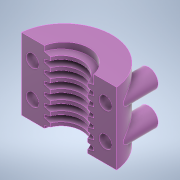
# Autodesk Inventor part: SpindleAdaptor_B_V2
Saved by Autodesk Inventor 2022.2 (Build 262287000, 287)
## iProperties
Created: 2022-11-20
Part Number: SpindleAdaptor_B_V2
Material: ABS Plastic
Document SubType Name: Modeling
Designer: jaege
Density: 1.06 g/cm^3
Appearance: Smooth - Purple
Mass: 4.16051 g
Surface Area: 27.1261 cm^2
Volume: 4.16051 cm^3
Author: jaege
Autodesk Inventor part; units mm, degrees
ref_plane "YZ Plane" through (0, 0, 0) normal (1, 0, 0) x (0, 1, 0)
ref_plane "XZ Plane" through (0, 0, 0) normal (0, 1, 0) x (-1, 0, 0)
ref_plane "XY Plane" through (0, 0, 0) normal (0, 0, 1) x (1, 0, 0)
sketch "Sketch1" plane through (0, 0, 0) normal (0, 1, 0) x (-1, 0, 0)
  circle A0 centre (0, 0) radius 10
  dimension "d0" = 20
  constraints: 1 centre point, 1 coincident
  measures "d0" diameter of A0
extrude "Extrusion1" add sketch "Sketch1" along normal blind 30
sketch "Sketch2" plane through (0, 30, 0) normal (0, 1, 0) x (1, 0, 0)
  circle A0 centre (0, 0) radius 5.25
  dimension "d3" = 10.5
  constraints: 1 centre point, 1 coincident
  measures "d3" diameter of A0
extrude "Extrusion2" cut sketch "Sketch2" against normal blind 15
sketch "Sketch3" plane through (0, 0, 0) normal (0, 0, 1) x (1, 0, 0)
  line L0 (10, 30) -> (-10, 30) projected
  line L1 (10, 0) -> (-10, 0) projected
  line L2 (-5.25, 15) -> (5.25, 15) projected
  line L3 (-5.25, 30) -> (5.25, 30) projected
  line L4 (-5.25, 30) -> (-5.25, 15) projected
  line L5 (5.25, 30) -> (5.25, 15) construction
  line L6 (-5.25, 15) -> (5.25, 15) projected
  line L7 (-4, 15) -> (4, 15) construction
  line L8 (4, 15) -> (4, 30) construction
  line L9 (4, 30) -> (-4, 30) construction
  line L10 (-4, 30) -> (-4, 15) construction
  line L11 (5.25, 30) -> (4, 29.6651)
  line L12 (2.634, 29.299) -> (4, 28.933) construction
  line L13 (4, 29.6651) -> (4, 28.933)
  line L14 (5.25, 28.5981) -> (5.25, 28)
  line L15 (5.25, 28) -> (4, 27.6651)
  line L16 (2.634, 27.299) -> (4, 26.933) construction
  line L17 (4, 29.6651) -> (2.634, 29.299) construction
  line L18 (4, 27.6651) -> (2.634, 27.299) construction
  line L19 (4, 28.933) -> (5.25, 28.5981)
  line L20 (4, 26.933) -> (5.25, 26.5981)
  line L21 (4, 27.6651) -> (4, 26.933)
  line L22 (5.25, 30) -> (5.25, 28.5981)
  line L23 (0, 30) -> (0, 15)
  point P0 (0, 0)
  point P1 (4, 29.299)
  dimension "d6" = 8
  dimension "d7" = 30
  dimension "d8" = 30
  dimension "d9" = 1.25
  dimension "d10" = 105
  dimension "d11" = 105
  dimension "d12" = 0.732
  dimension "d13" = 0.5981
  constraints: 34 end point, 9 point on line, 6 collinear, 3 midpoint, 2 parallel, 2 vertical, 1 horizontal, 1 perpendicular, 1 vertical alignment
  measures "d6" distance between parallel lines of L8 L10
  measures "d7" angle of L12 L11
  measures "d8" angle of L16 L15
  measures "d9" distance between parallel lines of L5 L13
  measures "d10" angle of L5 L11
  measures "d11" angle of L14 L15
  measures "d12" distance of L13.start L12.end
  measures "d13" distance of L14.start L14.end
coil "Coil1" sketch "Sketch3" operation add axis through (0, 30, 0) along (0, -1, 0) pitch 2 turns 7 hand right contours L22 L19 L13 L11
sketch "Sketch4" plane through (0, 0, 0) normal (0, -1, 0) x (1, 0, 0)
  circle A0 centre (0, 0) radius 2
  line L0 (-2, -2) -> (2, -2)
  line L1 (2, -2) -> (2, 1.5)
  line L2 (2, 1.5) -> (-2, 1.5)
  line L3 (-2, 1.5) -> (-2, -2)
  point P0 (1.3229, 1.5)
  point P1 (-1.3229, 1.5)
  dimension "d22" = 4
  dimension "d23" = 3.5
  constraints: 8 end point, 3 tangent, 2 parallel, 1 centre point, 1 coincident, 1 horizontal, 1 perpendicular
  measures "d22" diameter of A0
  measures "d23" distance of L0.end L1.end
extrude "Extrusion3" cut sketch "Sketch4" against normal blind 10 contours A0 L2 picked at (0.2249, -0.4939)
sketch "Sketch5" plane through (0, 0, 0) normal (0, 0, 1) x (1, 0, 0)
  line L0 (10, 30) -> (-10, 30) projected
  line L1 (-5.25, 15) -> (5.25, 15) projected
  line L2 (0, -6) -> (0, 36) projected
  line L3 (-7.625, 26) -> (-10, 26) construction
  line L4 (-7.625, 26) -> (-5.25, 26) construction
  line L5 (-5.25, 30) -> (-5.25, 15) projected
  line L6 (-10, 0) -> (-10, 30) projected
  circle A0 centre (-7.625, 19) radius 1.3375
  circle A1 centre (-7.625, 26) radius 1.3375
  circle A2 centre (7.625, 26) radius 1.3375
  circle A3 centre (7.625, 19) radius 1.3375
  point P0 (0, 0)
  point P1 (1.5921, 15)
  dimension "d26" = 4
  dimension "d27" = 4
  dimension "d28" = 2.675
  constraints: 4 centre point, 4 coincident, 4 end point, 4 vertical alignment, 3 equal radius, 2 horizontal, 2 horizontal alignment, 1 collinear, 1 symmetric about line
  measures "d26" distance from line of L0 L3.start
  measures "d27" distance from line of L1 point (-7.625, 19)
  measures "d28" diameter of A0
extrude "Extrusion4" cut sketch "Sketch5" along normal through all both and the other way through all contours A0 | A1 | A2 | A3
ref_plane "Work Plane1" through (0, 0, -10) normal (0, 0, -1) x (-1, 0, 0)
sketch "Sketch6" plane through (0, 0, -10) normal (0, 0, -1) x (-1, 0, 0)
  circle A0 centre (-7.625, 26) radius 1.3375
  line L0 (-10, 0) -> (-10, 30) projected
  line L1 (-5.25, 28.5981) -> (-5.25, 30) projected
  line L2 (10, 0) -> (10, 30) projected
  line L3 (10, 30) -> (-10, 30) projected
  line L4 (0, 30) -> (0, 0)
  line L5 (-7.625, 26) -> (-7.625, 29.0718) construction
  line L6 (-7.625, 29.0718) -> (-10, 29.0718) construction
  line L7 (-7.625, 29.0718) -> (-5.25, 29.0718) construction
  line L8 (-5.25, 15) -> (5.25, 15) projected
  circle A1 centre (-7.625, 19) radius 1.3375
  circle A2 centre (7.625, 19) radius 1.3375
  circle A3 centre (7.625, 26) radius 1.3375
  circle A4 centre (7.625, 19) radius 2
  circle A5 centre (7.625, 26) radius 2
  circle A6 centre (-7.625, 26) radius 2
  circle A7 centre (-7.625, 19) radius 2
  line L9 (-5.25, 28.5981) -> (-5.25, 0) construction
  line L10 (10, 0) -> (-10, 0) projected
  point P0 (-1.5921, 15)
  dimension "d31" = 2.675
  dimension "d32" = 4
  dimension "d33" = 4
  dimension "d34" = 4
  constraints: 10 end point, 8 centre point, 6 equal radius, 4 point on line, 3 coincident, 3 vertical, 2 horizontal alignment, 2 vertical alignment, 1 collinear, 1 midpoint, 1 perpendicular, 1 symmetric about line
  measures "d31" diameter of A0
  measures "d32" distance from line of L5.start L3
  measures "d33" distance from line of L8 A1.centre
  measures "d34" diameter of A7
ref_plane "Work Plane2" through (0, 0, 10) normal (0, 0, -1) x (-1, 0, 0)
extrude "Extrusion5" add sketch "Sketch6" against normal up to surface (20 mm away) contours A4 | A5 | A6 | A7
sketch "Sketch7" plane through (0, 30, 0) normal (0, 1, 0) x (1, 0, 0)
  circle A0 centre (0, 0) radius 10 projected
  line L0 (-14, -10) -> (14, -10) projected
  line L1 (-10, 0) -> (10, 0)
  line L2 (10, -10) -> (10, 0)
  line L3 (10, -10) -> (-10, -10)
  line L4 (-10, 0) -> (-10, -10)
  constraints: 8 end point, 2 point on circle, 2 point on line, 2 vertical, 1 horizontal, 1 midpoint
extrude "Extrusion6" cut sketch "Sketch7" against normal through all contours L2 L0 A0 | A0 L1 | A0 L0 L4 picked at (-2.0783, -2.6061)
sketch "Sketch8" plane through (-5.25, 15, 0) normal (0, 0, 1) x (1, 0, 0)
  line L0 (-4.75, -15) -> (-4.75, 15) projected
  line L1 (15.25, -15) -> (15.25, 15) projected
  line L2 (-4.75, 0) -> (15.25, 0)
  line L3 (15.25, 0) -> (15.25, -15)
  line L4 (15.25, -15) -> (-4.75, -15)
  line L5 (-4.75, -15) -> (-4.75, 0)
  point P0 (5.25, -15)
  constraints: 8 end point, 2 parallel, 1 horizontal, 1 midpoint, 1 perpendicular
extrude "Extrusion7" cut sketch "Sketch8" against normal through all
sketch "Sketch9" plane through (5.25, 30, 0) normal (0, 0, 1) x (1, 0, 0)
  line L0 (-15.25, -15) -> (-10.5, -15) projected
  line L1 (-10.5, -14.4019) -> (-10.5, -15) projected
  line L2 (-9.25, -13.3349) -> (-9.25, -14.067) projected
  line L3 (-10.5, -12.4019) -> (-10.5, -13) projected
  line L4 (-9.25, -11.3349) -> (-9.25, -12.067) projected
  line L5 (-10.5, -10.4019) -> (-10.5, -11) projected
  line L6 (-9.25, -9.3349) -> (-9.25, -10.067) projected
  line L7 (-10.5, -8.4019) -> (-10.5, -9) projected
  line L8 (-9.25, -7.3349) -> (-9.25, -8.067) projected
  line L9 (-10.5, -6.4019) -> (-10.5, -7) projected
  line L10 (-9.25, -5.3349) -> (-9.25, -6.067) projected
  line L11 (-10.5, -4.4019) -> (-10.5, -5) projected
  line L12 (-9.25, -3.3349) -> (-9.25, -4.067) projected
  line L13 (-10.5, -2.4019) -> (-10.5, -3) projected
  line L14 (-9.25, -1.3349) -> (-9.25, -2.067) projected
  line L15 (-10.5, 0) -> (-10.5, -1) projected
  line L16 (-15.25, 0) -> (-10.5, 0) projected
  line L17 (-15.25, -15) -> (-15.25, 0) projected
  circle A0 centre (-12.875, -4) radius 1.3375 projected
  circle A1 centre (-12.875, -11) radius 1.3375 projected
  circle A2 centre (2.375, -4) radius 1.3375 projected
  circle A3 centre (2.375, -11) radius 1.3375 projected
  line L18 (-1.25, -15) -> (4.75, -15) projected
  line L19 (4.75, -15) -> (4.75, 0) projected
  line L20 (0, 0) -> (4.75, 0) projected
  line L21 (0, -2) -> (0, 0) projected
  line L22 (-1.25, -3.067) -> (-1.25, -2.3349) projected
  line L23 (0, -4) -> (0, -3.4019) projected
  line L24 (-1.25, -5.067) -> (-1.25, -4.3349) projected
  line L25 (0, -6) -> (0, -5.4019) projected
  line L26 (-1.25, -7.067) -> (-1.25, -6.3349) projected
  line L27 (0, -8) -> (0, -7.4019) projected
  line L28 (-1.25, -9.067) -> (-1.25, -8.3349) projected
  line L29 (0, -10) -> (0, -9.4019) projected
  line L30 (-1.25, -11.067) -> (-1.25, -10.3349) projected
  line L31 (0, -12) -> (0, -11.4019) projected
  line L32 (-1.25, -13.067) -> (-1.25, -12.3349) projected
  line L33 (0, -14) -> (0, -13.4019) projected
  line L34 (0, -14) -> (-1.25, -14.3349) projected
  line L35 (-1.25, -14.3349) -> (-1.25, -15) projected
  line L36 (-15.25, 0) -> (4.75, 0)
  line L37 (4.75, 0) -> (4.75, -15)
  line L38 (4.75, -15) -> (-15.25, -15)
  line L39 (-15.25, -15) -> (-15.25, 0)
  point P0 (-5.25, -30)
  constraints: 8 end point, 2 parallel, 1 horizontal, 1 perpendicular, 26 other
extrude "Extrusion8" cut sketch "Sketch9" against normal blind 1 contours L17 L16 L36 L20 L19 L18 L38 L0 | A0 | A1 | A2 | A3
body "Solid1"
